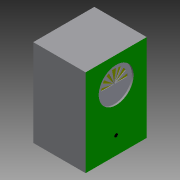
# Autodesk Inventor part: holder
Saved by Autodesk Inventor 2015 (Build 190159000, 159)
## iProperties
Created: 2017-04-05
Part Number: holder
Material: Generic
Document SubType Name: Modeling
Designer: Mohalla
Density: 1 g/cm^3
Appearance: Default
Mass: 52124.1 g
Surface Area: 8792.53 cm^2
Volume: 52124.1 cm^3
Author: Mohalla
Autodesk Inventor part; units mm, degrees
ref_plane "YZ Plane" through (0, 0, 0) normal (1, 0, 0) x (0, 1, 0)
ref_plane "XZ Plane" through (0, 0, 0) normal (0, 1, 0) x (-1, 0, 0)
ref_plane "XY Plane" through (0, 0, 0) normal (0, 0, 1) x (1, 0, 0)
sketch "Sketch1" plane through (0, 0, 0) normal (1, 0, 0) x (0, 1, 0)
  point P0 (0, 0)
sketch "Sketch2" plane through (0, 0, 0) normal (1, 0, 0) x (0, 1, 0)
  line L0 (500, 175) -> (0, 175)
  line L1 (0, 175) -> (0, -175)
  line L2 (0, -175) -> (500, -175)
  line L3 (500, -175) -> (500, 175)
  point P0 (0, 0)
  dimension "d0" = 500
  dimension "d1" = 350
  dimension "d2" = 175
  dimension "d3" = 500
  constraints: 8 end point, 2 parallel, 1 horizontal, 1 perpendicular
  measures "d0" distance of L0.start L0.end
  measures "d1" distance of L2.end L0.start
  measures "d2" distance from line of point (0, 0) L0
  measures "d3" distance from line of point (0, 0) L3
extrude "Extrusion1" add sketch "Sketch2" along normal blind 300
sketch "Sketch3" plane through (300, 0, 0) normal (1, 0, 0) x (0, 0, -1)
  circle A0 centre (0, 350) radius 100
  point P0 (0, 0)
  dimension "d6" = 200
  dimension "d7" = 350
  constraints: 1 centre point
  measures "d6" diameter of A0
  measures "d7" distance of point (0, 0) A0.centre
extrude "Extrusion2" cut sketch "Sketch3" against normal blind 10
sketch "Sketch6" plane through (290, 350, 0) normal (1, 0, 0) x (0, 0, -1)
  line L0 (-0.0604, -0.1466) -> (-75.0604, -0.1466)
  line L1 (-75.0604, -0.1466) -> (-0.0604, -0.1466)
  line L2 (-0.0604, -0.1466) -> (-73.5885, 14.6388)
  line L3 (-0.0604, -0.1466) -> (-67.2185, 33.4039)
  line L4 (-0.0604, -0.1466) -> (-58.5037, 46.9726)
  line L5 (-0.0604, -0.1466) -> (-45.1893, 59.847)
  line L6 (-0.0604, -0.1466) -> (-31.7085, 67.9287)
  line L7 (-0.0604, -0.1466) -> (-13.5499, 73.7038)
  line L8 (-0.0604, -0.1466) -> (11.8236, 73.9791)
  arc A0 (-73.5885, 14.6388) -> (-75.0604, -0.1466) centre (-37.9126, 3.6215) ccw
  arc A1 (-58.5037, 46.9726) -> (-67.2185, 33.4039) centre (-31.8389, 20.2637) ccw
  arc A2 (-31.7085, 67.9287) -> (-45.1893, 59.847) centre (-16.7307, 27.6606) ccw
  arc A3 (11.8236, 73.9791) -> (-13.5499, 73.7038) centre (-0.4454, 35.3353) ccw
  line L9 (-0.0604, -0.1466) -> (64.6218, 36.8812)
  line L10 (-0.0604, -0.1466) -> (51.5848, 53.6216)
  line L11 (-0.0604, -0.1466) -> (40.3954, 64.3692)
  line L12 (-0.0604, -0.1466) -> (23.8014, 71.9871)
  arc A4 (40.3954, 64.3692) -> (23.8014, 71.9871) centre (16.5753, 34.3639) ccw
  arc A5 (64.6218, 36.8812) -> (51.5848, 53.6216) centre (33.1363, 25.8077) ccw
  arc A6 (74.9396, -0.1466) -> (73.8878, 16.2903) centre (21.7524, 4.7019) ccw
  line L13 (73.8878, 16.2903) -> (-0.0604, -0.1466)
  line L14 (74.9396, -0.1466) -> (-0.0604, -0.1466)
  point P0 (0, -350)
  dimension "d18" = 75
  dimension "d20" = 11.37
  dimension "d21" = 75
  constraints: 30 end point, 14 point on circle, 7 centre point, 6 equal length, 2 horizontal, 1 collinear, 1 line through centre
  measures "d18" distance of L0.start L0.end
  measures "d20" angle of L2 L0
  measures "d21" distance of L0.start L14.start
extrude "Extrusion3" cut sketch "Sketch6" against normal blind 3
sketch "Sketch7" plane through (300, 0, 0) normal (1, 0, 0) x (0, 0, -1)
  circle A0 centre (0, 100) radius 10
  point P0 (0, 0)
  dimension "d24" = 100
  dimension "d25" = 20
  constraints: 1 centre point
  measures "d24" distance of point (0, 0) A0.centre
  measures "d25" diameter of A0
extrude "Extrusion4" cut sketch "Sketch7" against normal blind 150
equation "\"d21\" = d18"
body "Solid1"
